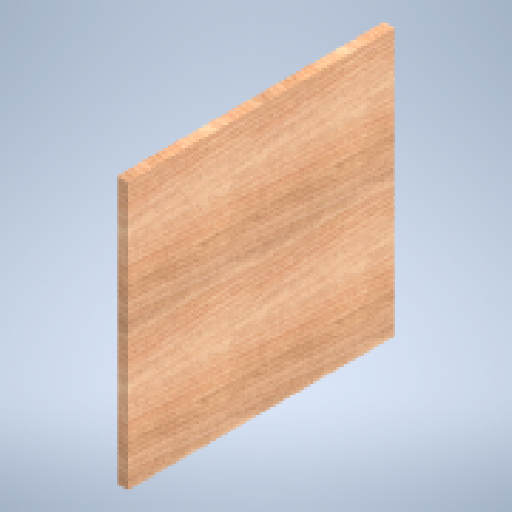
# Autodesk Inventor part: Sitzlehne
Saved by Autodesk Inventor 2024.4 (Build 284460000, 460)
## iProperties
Created: 2026-01-11
Part Number: Sitzlehne
Material: Holz (Birke)
Description: Sitzlehne
Document SubType Name: Modeling
Designer: julia
Mass: 2749.44 g
Surface Area: 5410.14 cm^2
Volume: 4998.97 cm^3
Density: 0.55 g/cm^3
Appearance: Birke - natur - poliert
DocNumber: Sitzlehne.ipt
Folder: I60-Konstruktion\I60-Gruppe-7\Sitz\
VDS_Category: Konstruktion
Masse[kg]: 2,749 kg
Autodesk Inventor part; units mm, degrees
ref_plane "YZ Plane" through (0, 0, 0) normal (1, 0, 0) x (0, 1, 0)
ref_plane "XZ Plane" through (0, 0, 0) normal (0, 1, 0) x (-1, 0, 0)
ref_plane "XY Plane" through (0, 0, 0) normal (0, 0, 1) x (1, 0, 0)
sketch "Skizze1" plane through (0, 0, 0) normal (1, 0, 0) x (0, 1, 0)
  line L0 (-250, 250) -> (250, 250)
  line L1 (250, 250) -> (250, -250)
  line L2 (250, -250) -> (-250, -250)
  line L3 (-250, -250) -> (-250, 250)
  line L4 (-250, 250) -> (250, -250) construction
  line L5 (250, 250) -> (-250, -250) construction
  point P0 (0, 0)
  dimension "d0" = 500
  dimension "d1" = 500
  constraints: 12 end point, 2 midpoint, 2 parallel, 1 horizontal, 1 perpendicular
  measures "d0" distance of L1.end L2.end
  measures "d1" distance of L0.end L1.end
extrude "Extrusion1" add sketch "Skizze1" along normal blind 20
sketch "Skizze4" plane through (0, 250, 250) normal (0, 1, 0) x (1, 0, 0)
  line L0 (20, 500) -> (8, 500)
  line L1 (0, 500) -> (20, 500) projected
  line L2 (8, 500) -> (8, 415)
  line L3 (8, 415) -> (8, 403)
  line L4 (8, 403) -> (8, 367)
  line L5 (0, 500) -> (0, 0) projected
  line L6 (20, 500) -> (20, 0) projected
  line L7 (20, 0) -> (8, 0)
  line L8 (0, 0) -> (20, 0) projected
  line L9 (8, 0) -> (8, 85)
  line L10 (8, 85) -> (8, 97)
  line L11 (8, 97) -> (8, 133)
  point P0 (0, 250)
  dimension "d37" = 85
  dimension "d38" = 12
  dimension "d39" = 36
  dimension "d41" = 12
  dimension "d42" = 85
  dimension "d43" = 12
  dimension "d44" = 36
  constraints: 16 end point, 6 point on line, 2 perpendicular
  measures "d37" distance of L0.end L2.end
  measures "d38" distance of L2.end L3.end
  measures "d39" distance of L3.end L4.end
  measures "d41" distance of L6.end L7.end
  measures "d42" distance of L7.end L9.end
  measures "d43" distance of L9.end L10.end
  measures "d44" distance of L10.end L11.end
hole "Bohrung1" at (8, 250, -153) at (8, 250, -117) at (8, 250, 153) at (8, 250, 117) direction (0, -1, 0) diameter 4 depth 20 tip angle 118
